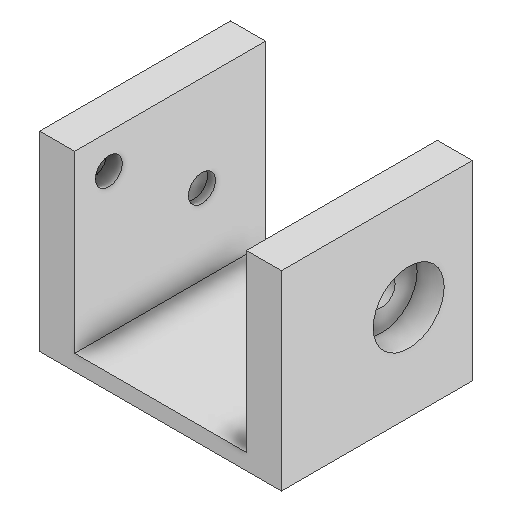
# Autodesk Inventor part: Base
Saved by Autodesk Inventor 2026.2 (Build 302298000, 298)
## iProperties
Created: 2025-12-27
Part Number: Base
Material: 一般
Document SubType Name: Modeling
Designer: Hsiangyu
Density: 1 g/cm^3
Appearance: 預設
Author: Hsiangyu
Autodesk Inventor part; units mm, degrees
ref_plane "YZ Plane" through (0, 0, 0) normal (1, 0, 0) x (0, 1, 0)
ref_plane "XZ Plane" through (0, 0, 0) normal (0, 1, 0) x (-1, 0, 0)
ref_plane "XY Plane" through (0, 0, 0) normal (0, 0, 1) x (1, 0, 0)
sketch "草圖1" plane through (0, 0, 0) normal (0, 1, 0) x (-1, 0, 0)
  line L0 (-38, 30) -> (38, 30)
  line L1 (38, 30) -> (38, -30)
  line L2 (38, -30) -> (-38, -30)
  line L3 (-38, -30) -> (-38, 30)
  point P0 (0, 0)
  point P1 (0, -30)
  point P2 (38, 0)
  dimension "d0" = 60
  dimension "d1" = 76
  constraints: 8 end point, 2 midpoint, 2 parallel, 1 horizontal, 1 horizontal alignment, 1 perpendicular, 1 vertical alignment
  measures "d0" distance of L0.end L1.end
  measures "d1" distance of L1.end L2.end
extrude "擠出1" add sketch "草圖1" along normal blind 5
sketch "草圖2" plane through (0, 5, 0) normal (0, 1, 0) x (1, 0, 0)
  line L0 (38, 30) -> (-38, 30) projected
  line L1 (-38, 30) -> (-38, -30) projected
  line L2 (-38, -30) -> (38, -30) projected
  line L3 (38, -30) -> (38, 30) projected
  line L4 (-27, 30) -> (-27, -30)
  line L5 (27, -30) -> (27, 30)
  point P0 (0, 0)
  dimension "d4" = 11
  dimension "d5" = 11
  constraints: 4 end point, 4 point on line, 2 perpendicular
  measures "d4" distance between parallel lines of L1 L4
  measures "d5" distance between parallel lines of L3 L5
extrude "擠出2" add sketch "草圖2" along normal blind 55 contours L3 L2 L5 L0 | L4 L2 L1 L0
sketch "草圖3" plane through (38, 0, 30) normal (1, 0, 0) x (0, 0, -1)
  line L0 (60, 0) -> (60, 60) projected
  line L1 (0, 5) -> (60, 5) projected
  circle A0 centre (40, 30) radius 11.2
  line L2 (10.7467, 49.2158) -> (40, 30)
  point P0 (30, 0)
  dimension "d8" = 22.4
  dimension "d9" = 25
  dimension "d10" = 20
  dimension "d25" = 35
  dimension "d26" = 33.3
  constraints: 2 end point, 1 centre point, 1 coincident
  measures "d8" diameter of A0
  measures "d9" distance from line of A0.centre L1
  measures "d10" distance from line of L0 A0.centre
  measures "d25" distance of L2.start L2.end
  measures "d26" angle of L1 L2
sketch "草圖4" plane through (-38, 0, -30) normal (-1, 0, 0) x (0, 0, 1)
  line L0 (0, 0) -> (0, 60) projected
  line L1 (0, 5) -> (60, 5) projected
  circle A0 centre (20, 30) radius 11.2
  line L2 (20, 30) -> (49.2533, 49.2158)
  point P0 (30, 0)
  dimension "d13" = 22.4
  dimension "d14" = 25
  dimension "d15" = 20
  dimension "d41" = 35
  dimension "d42" = 33.3
  constraints: 2 end point, 1 centre point
  measures "d13" diameter of A0
  measures "d14" distance from line of L1 L2.start
  measures "d15" distance from line of L0 L2.start
  measures "d41" distance of L2.start L2.end
  measures "d42" angle of L1 L2
hole "孔1" at (38, 30, -10) direction (-1, 0, 0) diameter 8.5 end through all counterbore diameter 22.3 counterbore depth 8.5
hole "孔2" at (-38, 30, -10) direction (1, 0, 0) diameter 8.5 end through all counterbore diameter 22.3 counterbore depth 8.5
hole "孔4" at (-38, 49.2158, 19.2533) direction (1, 0, 0) diameter 8.5 depth 11 counterbore diameter 12.3 counterbore depth 6
equation "\"d13\" = d8"
equation "\"d14\" = d9"
equation "\"d15\" = d10"
